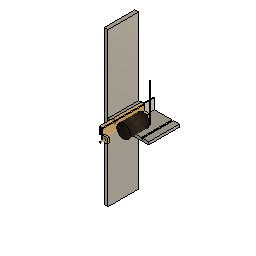
fusion360-archive-file (Autodesk Fusion 360 design; units mm, degrees)
Autodesk Fusion 360 part; units mm, degrees
sketch "basicTable" plane through (0, 0, 0) normal (0, 0, 1) x (1, 0, 0) in component "table"
  line L0 (0, 0) -> (539.75, 0)
  line L1 (539.75, 0) -> (539.75, 406.4)
  line L2 (539.75, 406.4) -> (0, 406.4)
  line L3 (0, 406.4) -> (0, 0)
  dimension "d40" = 539.75
  dimension "d41" = 406.4
  constraint horizontal L0
  constraint vertical L1
  constraint horizontal L2
  constraint vertical L3
  constraint coincident L0.start L3.end
  measures "d40" distance of L0.start L0.end
  measures "d41" distance of L0.start L2.end
extrude "ExtrudeTableThickness" add sketch "basicTable" along normal blind 36.5125 makes body 1 in component "table"
sketch "miterOutline and Blade Placement" plane through (0, 0, 36.5125) normal (0, 0, 1) x (-1, 0, 0) in component "table"
  line L0 (0, -406.4) -> (0, 0)
  line L1 (0, 0) -> (-539.75, 0)
  line L2 (-539.75, 0) -> (-539.75, -406.4)
  line L3 (-539.75, -406.4) -> (0, -406.4)
  line L4 (-441.325, -406.4) -> (-460.375, -406.4)
  line L5 (-460.375, -406.4) -> (-460.375, 0)
  line L6 (-460.375, 0) -> (-441.325, 0)
  line L7 (-441.325, 0) -> (-441.325, -406.4)
  line L8 (-352.425, -406.4) -> (-352.425, 0) construction
  line L9 (-441.325, -203.2) -> (0, -203.2) construction
  point P0 (-352.425, -203.2)
  dimension "d44" = 79.375
  dimension "d45" = 19.05
  dimension "d46" = 88.9
  dimension "d47" = 203.2
  constraint horizontal L4
  constraint vertical L5
  constraint horizontal L6
  constraint vertical L7
  constraint coincident L1 L5.end
  constraint coincident L3 L4.start
  constraint coincident L3 L8.start
  constraint coincident L1 L8.end
  constraint perpendicular L1 L8
  constraint coincident L7 L9.start
  constraint coincident L0 L9.end
  constraint perpendicular L0 L9
  constraint midpoint L8 P0
  measures "d44" distance of L2 L5
  measures "d45" distance of L5 L7
  measures "d46" distance of L7 L8
  measures "d47" distance of L1 L9
extrude "ExtrudeMiterSlot" cut sketch "miterOutline and Blade Placement" against normal blind 12.7 contours L1 L3 L4 L5 L6 L7 bodies 1 in component "table"
sketch "Sketch1" plane through (0, 0, 36.5125) normal (0, 0, 1) x (-1, 0, 0) in component "BandsawBlade"
  line L0 (-351.6312, -196.85) -> (-353.2187, -196.85)
  line L1 (-353.2187, -196.85) -> (-353.2187, -209.55)
  line L2 (-353.2187, -209.55) -> (-351.6312, -209.55)
  line L3 (-351.6312, -209.55) -> (-351.6312, -196.85)
  line L4 (-351.6312, -196.85) -> (-353.2187, -209.55) construction
  line L5 (-353.2187, -196.85) -> (-351.6312, -209.55) construction
  point P0 (-352.425, -203.2)
  point P1 (-352.425, -203.2)
  dimension "d76" = 1.5875
  dimension "d77" = 12.7
  constraint horizontal L0
  constraint perpendicular L0 L1
  constraint parallel L0 L2
  constraint parallel L1 L3
  constraint coincident L4 P1
  constraint coincident L5 P1
  constraint coincident P1 P0
  measures "d76" distance of L1.end L2.end
  measures "d77" distance of L0.end L1.end
extrude "Extrude1" add sketch "Sketch1" along normal blind 508 separate body makes body 2 in component "BandsawBlade"
sketch "logCylinder" plane through (0, 0, 0) normal (0, 1, 0) x (1, 0, 0) in component "Log"
  circle A0 centre (169.0248, -125.4125) radius 88.9
  line L0 (0, -36.5125) -> (441.325, -36.5125)
  point P0 (169.0248, -125.4125)
  point P1 (139.7, -76.2)
  dimension "d204" = 177.8
  constraint tangent A0 L0
  constraint coincident P0 A0.centre
  measures "d204" diameter of A0
extrude "Extrude1'" add sketch "logCylinder" along normal blind 254 separate body makes body 3 in component "Log"
sketch "Sketch2" plane through (0, 0, 36.5125) normal (0, 0, 1) x (-1, 0, 0)
  line L0 (-441.325, 0) -> (-441.325, -406.4)
  line L1 (-441.325, -406.4) -> (0, -406.4)
  line L2 (0, -406.4) -> (0, 0)
  line L3 (0, 0) -> (-441.325, 0)
sketch "Sketch3" plane through (0, 0, 0) normal (0, -1, 0) x (1, 0, 0)
  line L0 (460.375, 36.5125) -> (460.375, 23.8125)
  line L1 (460.375, 23.8125) -> (441.325, 23.8125)
  line L2 (441.325, 23.8125) -> (441.325, 36.5125)
  line L3 (441.325, 36.5125) -> (0, 36.5125)
  line L4 (0, 36.5125) -> (0, 0)
  line L5 (0, 0) -> (539.75, 0)
  line L6 (539.75, 0) -> (539.75, 36.5125)
  line L7 (539.75, 36.5125) -> (460.375, 36.5125)
sketch "Sketch1 (2)" plane through (0, 0, 0) normal (0, -1, 0) x (1, 0, 0) in component "Fence"
  line L0 (441.325, 36.5125) -> (0, 36.5125)
  line L1 (38.1, 36.5125) -> (0, 36.5125)
  line L2 (38.1, 36.5125) -> (38.1, 176.2125)
  line L3 (38.1, 176.2125) -> (25.4, 176.2125)
  line L4 (25.4, 176.2125) -> (25.4, 100.0125)
  line L5 (25.4, 100.0125) -> (0, 100.0125)
  line L6 (0, 100.0125) -> (0, 36.5125)
  point P0 (0, 36.5125)
  dimension "d255" = 38.1
  dimension "d256" = 139.7
  dimension "d257" = 12.7
  dimension "d258" = 76.2
  dimension "d259" = 25.4
  constraint coincident L0 L1.start
  constraint coincident P0 L0.end
  constraint perpendicular L0 L2
  constraint horizontal L3
  constraint perpendicular L3 L4
  constraint horizontal L5
  measures "d255" distance of L1.start P0
  measures "d256" distance of L1.start L2.end
  measures "d257" distance of L2.end L3.end
  measures "d258" distance of L3.end L4.end
  measures "d259" distance of L4.end L5.end
extrude "Extrude1''" add sketch "Sketch1 (2)" against normal blind 406.4 separate body makes body 4 in component "Fence"
sketch "leftJigPlate" plane through (0, 0, 0) normal (0, -1, 0) x (1, 0, 0) in component "jig"
  line L0 (25.4, 100.0125) -> (12.7, 100.0125)
  line L1 (12.7, 100.0125) -> (12.7, 176.2125)
  line L2 (12.7, 176.2125) -> (25.4, 176.2125)
  line L3 (25.4, 176.2125) -> (25.4, 100.0125)
  point P0 (25.4, 100.0125)
  dimension "d263" = 12.7
  dimension "d264" = 76.2
  constraint horizontal L0
  constraint vertical L1
  constraint horizontal L2
  constraint vertical L3
  constraint coincident P0 L0.start
  measures "d263" distance of P0 L0.end
  measures "d264" distance of P0 L2.end
sketch "topJigPlate" plane through (0, 0, 0) normal (0, -1, 0) x (1, 0, 0) in component "jig"
  line L0 (12.7, 176.2125) -> (50.8, 176.2125)
  line L1 (50.8, 176.2125) -> (50.8, 188.9125)
  line L2 (50.8, 188.9125) -> (12.7, 188.9125)
  line L3 (12.7, 188.9125) -> (12.7, 176.2125)
  point P0 (12.7, 176.2125)
  dimension "d265" = 38.1
  dimension "d266" = 12.7
  constraint horizontal L0
  constraint vertical L1
  constraint horizontal L2
  constraint vertical L3
  constraint coincident P0 L0.start
  measures "d265" distance of P0 L0.end
  measures "d266" distance of P0 L2.end
sketch "rightJigPlate" plane through (0, 0, 0) normal (0, -1, 0) x (1, 0, 0) in component "jig"
  line L0 (38.1, 36.5125) -> (38.1, 176.2125)
  line L1 (38.1, 176.2125) -> (25.4, 176.2125)
  line L2 (25.4, 176.2125) -> (25.4, 100.0125)
  line L3 (25.4, 100.0125) -> (0, 100.0125)
  line L4 (0, 100.0125) -> (0, 36.5125)
  line L5 (0, 36.5125) -> (38.1, 36.5125)
  line L6 (50.8, 176.2125) -> (38.1, 176.2125)
  line L7 (38.1, 176.2125) -> (38.1, 36.5125)
  line L8 (38.1, 36.5125) -> (50.8, 36.5125)
  line L9 (50.8, 36.5125) -> (50.8, 176.2125)
  point P0 (50.8, 176.2125)
  constraint horizontal L6
  constraint vertical L7
  constraint horizontal L8
  constraint vertical L9
  constraint coincident L0.start L5.end
  constraint coincident P0 L6.start
extrude "Extrude1'''" add sketch "leftJigPlate" against normal blind 558.8 separate body makes body 5 in component "jig"
extrude "Extrude2" add sketch "topJigPlate" against normal blind 558.8 separate body makes body 6 in component "jig"
extrude "Extrude3" add sketch "rightJigPlate" against normal blind 558.8 separate body contours L0 L6 L7 L8 L9 makes body 7 in component "jig"
sketch "frontJigBlock" plane through (0, 0, 0) normal (0, -1, 0) x (1, 0, 0) in component "jig"
  line L0 (50.8, 36.5125) -> (50.8, 176.2125)
  line L1 (50.8, 176.2125) -> (38.1, 176.2125)
  line L2 (38.1, 176.2125) -> (38.1, 36.5125)
  line L3 (38.1, 36.5125) -> (50.8, 36.5125)
  line L4 (50.8, 36.5125) -> (120.65, 36.5125)
  line L5 (120.65, 36.5125) -> (120.65, 106.3625)
  line L6 (120.65, 106.3625) -> (50.8, 106.3625)
  line L7 (50.8, 106.3625) -> (50.8, 36.5125)
  dimension "d274" = 69.85
  dimension "d275" = 69.85
  constraint horizontal L4
  constraint vertical L5
  constraint horizontal L6
  constraint vertical L7
  constraint coincident L0.start L3.end
  measures "d274" distance of L0.start L4.end
  measures "d275" distance of L0.start L6.end
sketch "backJigBlock" plane through (0, 558.8, 0) normal (0, 1, 0) x (-1, 0, 0) in component "jig"
  line L0 (-50.8, 176.2125) -> (-50.8, 36.5125)
  line L1 (-50.8, 36.5125) -> (-38.1, 36.5125)
  line L2 (-38.1, 36.5125) -> (-38.1, 176.2125)
  line L3 (-38.1, 176.2125) -> (-50.8, 176.2125)
  line L4 (-120.65, 36.5125) -> (-50.8, 36.5125)
  line L5 (-50.8, 106.3625) -> (-120.65, 106.3625)
  line L6 (-50.8, 36.5125) -> (-50.8, 106.3625)
  line L7 (-120.65, 36.5125) -> (-120.65, 106.3625)
  dimension "d277" = 69.85
  dimension "d278" = 69.85
  constraint horizontal L4
  constraint vertical L6
  constraint horizontal L5
  constraint perpendicular L5 L7
  constraint coincident L0.end L1.start
  measures "d277" distance of L4.start L0.end
  measures "d278" distance of L4.start L5.end
extrude "Extrude4" add sketch "frontJigBlock" against normal blind 25.4 separate body contours L0 L4 L5 L6 L7 makes body 8 in component "jig"
extrude "Extrude5" add sketch "backJigBlock" against normal blind 25.4 separate body contours L0 L4 L5 L6 L7 makes body 9 in component "jig"
copy_body "Body->Comp1" bodies 5 removing the originals makes body 10 in component "leftJigPlate"
copy_body "Body->Comp2" bodies 8 removing the originals makes body 11 in component "frontJigPlate"
copy_body "Body->Comp3" bodies 6 removing the originals makes body 12 in component "topJigPlate"
copy_body "Body->Comp4" bodies 7 removing the originals makes body 13 in component "rightJigPlate"
copy_body "Body->Comp5" bodies 9 removing the originals makes body 14 in component "rearJigPlate"
sketch "Sketch1 (3)" plane through (0, 533.4, 0) normal (0, -1, 0) x (1, 0, 0) in component "rearJigPlate"
  line L0 (50.8, 106.3625) -> (50.8, 36.5125)
  line L1 (50.8, 36.5125) -> (120.65, 36.5125)
  line L2 (120.65, 36.5125) -> (120.65, 106.3625)
  line L3 (120.65, 106.3625) -> (50.8, 106.3625)
  line L4 (50.8, 71.4375) -> (120.65, 71.4375) construction
  line L5 (85.725, 106.3625) -> (85.725, 36.5125) construction
  circle A0 centre (85.725, 71.4375) radius 9.525
  dimension "d283" = 19.05
  constraint midpoint L0 L4.start
  constraint midpoint L2 L4.end
  constraint midpoint L3 L5.start
  constraint midpoint L1 L5.end
  constraint midpoint L4 A0.centre
  measures "d283" diameter of A0
extrude "Extrude1''''" cut sketch "Sketch1 (3)" against normal blind 12.7 contours A0 bodies 14 in component "rearJigPlate"
sketch "Sketch1 (4)" plane through (0, 0, 0) normal (0, -1, 0) x (1, 0, 0) in component "frontJigPlate"
  line L0 (50.8, 106.3625) -> (50.8, 36.5125)
  line L1 (120.65, 36.5125) -> (120.65, 106.3625)
  line L2 (50.8, 71.4375) -> (120.65, 71.4375) construction
  line L3 (50.8, 36.5125) -> (120.65, 36.5125)
  line L4 (120.65, 106.3625) -> (50.8, 106.3625)
  line L5 (85.725, 36.5125) -> (85.725, 106.3625) construction
  circle A0 centre (85.725, 71.4375) radius 9.525
  dimension "d286" = 19.05
  constraint midpoint L0 L2.start
  constraint midpoint L1 L2.end
  constraint midpoint L3 L5.start
  constraint midpoint L4 L5.end
  constraint midpoint L5 A0.centre
  measures "d286" diameter of A0
extrude "Extrude1'''''" cut sketch "Sketch1 (4)" against normal blind 25.4 contours A0 bodies 11 in component "frontJigPlate"
extrude "Extrude1''''''" add 1 faces at (86.3729, 546.1, 77.328) along direction (0, -1, 0) blind 609.6 separate body on bodies 14 makes body 15 in component "pipe"
sketch "centerPointTangentLine" plane through (0, 0, 0) normal (0, -1, 0) x (1, 0, 0) in component "Log"
  circle A0 centre (169.0248, 125.4125) radius 88.9
  line L0 (169.0248, 125.4125) -> (169.0248, 36.5125) construction
  line L1 (169.0248, 71.4375) -> (98.3855, 71.4375) construction
  point P0 (169.0248, 125.4125)
  point P1 (169.0248, 71.4375)
  dimension "d344" = 34.925
  constraint coincident P0 A0.centre
  constraint coincident A0 L0.end
  constraint vertical L0
  constraint coincident L0 P1
  constraint coincident P1 L1.start
  constraint coincident A0 L1.end
  constraint perpendicular L0 L1
  measures "d344" distance of L0.end P1
sketch "Sketch1 (5)" plane through (0, -63.5, 0) normal (0, -1, 0) x (1, 0, 0) in component "pipe"
  circle A0 centre (85.725, 71.4375) radius 9.525
  line L0 (85.725, 71.4375) -> (95.25, 71.4375) construction
  point P0 (85.725, 71.4375)
  constraint coincident P0 A0.centre
  constraint coincident A0 L0.end
  constraint horizontal L0
sketch "Sketch1 (6)" plane through (0, 0, 0) normal (-1, 0, 0) x (0, -1, 0) in component "bandsawFrame"
  line L0 (-406.4, 0) -> (0, 0)
  line L1 (0, 0) -> (0, 36.5125)
  line L2 (0, 36.5125) -> (-406.4, 36.5125)
  line L3 (-406.4, 36.5125) -> (-406.4, 0)
  line L4 (-406.4, 36.5125) -> (0, 36.5125)
  line L5 (0, 36.5125) -> (0, 1052.5125)
  line L6 (0, 1052.5125) -> (-406.4, 1052.5125)
  line L7 (-406.4, 1052.5125) -> (-406.4, 36.5125)
  line L8 (-406.4, 36.5125) -> (0, 36.5125)
  line L9 (0, 36.5125) -> (0, -979.4875)
  line L10 (0, -979.4875) -> (-406.4, -979.4875)
  line L11 (-406.4, -979.4875) -> (-406.4, 36.5125)
  dimension "d359" = 406.4
  dimension "d360" = 1016
  dimension "d361" = 406.4
  dimension "d362" = 1016
  constraint horizontal L4
  constraint vertical L5
  constraint horizontal L6
  constraint vertical L7
  constraint coincident L2.end L3.start
  constraint horizontal L8
  constraint vertical L9
  constraint horizontal L10
  constraint vertical L11
  measures "d359" distance of L5 L7
  measures "d360" distance of L4 L6
  measures "d361" distance of L9 L11
  measures "d362" distance of L8 L10
extrude "Extrude1'''''''" add sketch "Sketch1 (6)" along normal blind 50.8 separate body makes body 16 in component "bandsawFrame"
component "table" placed x (1, 0, 0) y (0, 1, 0) z (0, 0, 1) at (0, 0, 0)
component "BandsawBlade" placed x (1, 0, 0) y (0, 1, 0) z (0, 0, 1) at (0, 0, 0)
component "Log" placed x (1, 0, 0) y (0, 1, 0) z (0, 0, 1) at (162.5911, 83.5073, 0)
component "Fence" placed x (1, 0, 0) y (0, 1, 0) z (0, 0, 1) at (165.7266, 0, 0)
component "jig" placed x (1, 0, 0) y (0, 1, 0) z (0, 0, 1) at (165.7266, 58.1073, 0)
component "pipe" placed x (1, 0, 0) y (0, 1, 0) z (0, 0, 1) at (165.7266, 58.1073, 0)
component "bandsawFrame" placed x (1, 0, 0) y (0, 1, 0) z (0, 0, 1) at (0, 0, 0)
component "leftJigPlate" placed x (1, 0, 0) y (0, 1, 0) z (0, 0, 1) at (0, 0, 0) in component "jig"
component "frontJigPlate" placed x (1, 0, 0) y (0, 1, 0) z (0, 0, 1) at (0, 0, 0) in component "jig"
component "topJigPlate" placed x (1, 0, 0) y (0, 1, 0) z (0, 0, 1) at (0, 0, 0) in component "jig"
component "rightJigPlate" placed x (1, 0, 0) y (0, 1, 0) z (0, 0, 1) at (0, 0, 0) in component "jig"
component "rearJigPlate" placed x (1, 0, 0) y (0, 1, 0) z (0, 0, 1) at (0, 0, 0) in component "jig"
equation "tableWidth = 21.25 in"
equation "tableDepth = 16 in"
equation "miterWidth = 0.75 in"
equation "miterHeight = 0.5 in"
equation "tableThickness = 1 in + ( ( 7 / 16 ) * 1 in )"
equation "MiterEdgeToRightTableEdge = 3 in + ( ( 1 / 8 ) * 1 in )"
equation "MiterEdgeToBlade = 3.5 in"
equation "bladeDistanceFromFront = 8 in"
equation "d40 = tableWidth"
equation "d41 = tableDepth"
equation "d42 = tableThickness"
equation "d44 = MiterEdgeToRightTableEdge"
equation "d45 = miterWidth"
equation "d46 = MiterEdgeToBlade"
equation "d47 = bladeDistanceFromFront"
equation "d48 = -miterHeight"
equation "bladeThickness = ( 1 / 16 ) * 1 in"
equation "bladeWidth = ( 1 / 2 ) * 1 in"
equation "bladeHeight = 20 in"
equation "d76 = bladeThickness"
equation "d77 = bladeWidth"
equation "d78 = bladeHeight"
equation "d204 = logDiameter"
equation "logDiameter = 7 in"
equation "logDepth = 10 in"
equation "d207 = logDepth"
equation "d243 = logDiameter / 2"
equation "d245 = logDepth / 2"
equation "d260 = -tableDepth"
equation "d266 = ( 1 / 2 ) * 1 in"
equation "jigDepth = tableDepth + 6 in"
equation "d268 = -jigDepth"
equation "d270 = -jigDepth"
equation "d272 = -jigDepth"
equation "d274 = jigBlockWidth"
equation "d275 = jigBlockHeight"
equation "jigBlockDepth = 1 in"
equation "d277 = jigBlockWidth"
equation "d278 = jigBlockHeight"
equation "d279 = -jigBlockDepth"
equation "d281 = -jigBlockDepth"
equation "d283 = ( 3 / 4 ) * 1 in"
equation "d284 = -jigBlockDepth / 2"
equation "d286 = ( 3 / 4 ) * 1 in"
equation "d287 = -jigBlockDepth"
equation "d313 = pipeLength"
equation "pipeLength = 24 in"
equation "d333 = logDiameter / 2"
equation "d344 = jigBlockHeight / 2"
equation "jigBlockWidth = 2.75 in"
equation "jigBlockHeight = 2.75 in"
equation "d359 = tableDepth"
equation "d361 = tableDepth"
named bodies: "leftJigPlate", "rightJigPlate", "topJigPlate", "frontJigPlate", "rearJigPlate"
